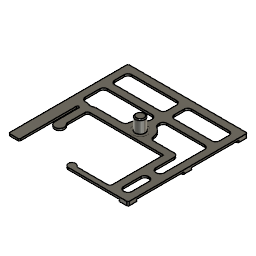
StentorCam Base (Autodesk Fusion 360 design; units mm, degrees)
Autodesk Fusion 360 part; units mm, degrees
note: some values were not read from the file. Set by a fixed rule: which sketch regions a step uses.
sketch "Sketch1" plane through (0, 0, 0) normal (0, 0, 1) x (1, 0, 0)
  line L0 (0, 0) -> (235, 0)
  line L1 (235, 0) -> (235, 235)
  line L2 (235, 235) -> (0, 235)
  line L3 (0, 235) -> (0, 0)
  line L4 (42.1, 114.8) -> (192.9, 114.8)
  line L5 (192.9, 114.8) -> (192.9, 10.2)
  line L6 (192.9, 10.2) -> (42.1, 10.2)
  line L7 (42.1, 10.2) -> (42.1, 114.8)
  line L8 (42.1, 114.8) -> (192.9, 10.2) construction
  line L9 (192.9, 114.8) -> (42.1, 10.2) construction
  circle A0 centre (125, 135) radius 10
  line L10 (125, 125) -> (117.5, 125) construction
  line L11 (117.5, 125) -> (117.5, 0) construction
  line L12 (-5, 240) -> (-5, -5)
  line L13 (-5, -5) -> (240, -5)
  line L14 (240, -5) -> (240, 240)
  line L15 (240, 240) -> (-5, 240)
  line L16 (117.5, 0) -> (117.5, -5) construction
  line L17 (110, -5) -> (125, -5)
  arc A1 (125, -5) -> (125, 0) centre (125, -2.5) ccw
  line L18 (125, 0) -> (110, 0)
  arc A2 (110, 0) -> (110, -5) centre (110, -2.5) ccw
  line L19 (110, -2.5) -> (125, -2.5) construction
  arc A3 (12.5, -5) -> (12.5, 0) centre (12.5, -2.5) ccw
  arc A4 (-2.5, 0) -> (-2.5, -5) centre (-2.5, -2.5) ccw
  arc A5 (237.5, -5) -> (237.5, 0) centre (237.5, -2.5) ccw
  arc A6 (222.5, 0) -> (222.5, -5) centre (222.5, -2.5) ccw
  line L20 (0, 117.5) -> (235, 117.5) construction
  circle A7 centre (125, 135) radius 15
  circle A8 centre (32.1, 62.5) radius 10
  line L21 (37.1, 62.5) -> (22.1, 62.5)
  line L22 (22.1, 62.5) -> (22.1, 114.8)
  line L23 (22.1, 114.8) -> (37.1, 114.8)
  line L24 (37.1, 114.8) -> (37.1, 62.5)
  line L25 (42.1, 114.8) -> (17.1, 114.8)
  line L26 (17.1, 114.8) -> (17.1, 10.2)
  line L27 (17.1, 10.2) -> (42.1, 10.2)
  line L28 (42.1, 10.2) -> (42.1, 114.8)
  circle A9 centre (117.5, 2.6) radius 7.6
  line L29 (117.5, -5) -> (17.1, -5)
  line L30 (17.1, -5) -> (17.1, 5.2)
  line L31 (17.1, 5.2) -> (117.5, 5.2)
  line L32 (117.5, 5.2) -> (117.5, -5)
  line L33 (192.9, 10.2) -> (17.1, 10.2)
  line L34 (17.1, 10.2) -> (17.1, 5.2)
  line L35 (17.1, 5.2) -> (192.9, 5.2)
  line L36 (192.9, 5.2) -> (192.9, 10.2)
  line L37 (192.9, 5.2) -> (192.9, -5)
  line L38 (17.1, 114.8) -> (-5, 114.8)
  arc A10 (235, -2.5) -> (240, -2.5) centre (237.5, -2.5) ccw
  arc A11 (240, 12.5) -> (235, 12.5) centre (237.5, 12.5) ccw
  arc A12 (235, 110) -> (240, 110) centre (237.5, 110) ccw
  arc A13 (240, 125) -> (235, 125) centre (237.5, 125) ccw
  arc A14 (235, 222.5) -> (240, 222.5) centre (237.5, 222.5) ccw
  arc A15 (240, 237.5) -> (235, 237.5) centre (237.5, 237.5) ccw
  arc A16 (237.5, 235) -> (237.5, 240) centre (237.5, 237.5) ccw
  arc A17 (222.5, 240) -> (222.5, 235) centre (222.5, 237.5) ccw
  arc A18 (125, 235) -> (125, 240) centre (125, 237.5) ccw
  arc A19 (110, 240) -> (110, 235) centre (110, 237.5) ccw
  arc A20 (12.5, 235) -> (12.5, 240) centre (12.5, 237.5) ccw
  arc A21 (-2.5, 240) -> (-2.5, 235) centre (-2.5, 237.5) ccw
  arc A22 (0, 237.5) -> (-5, 237.5) centre (-2.5, 237.5) ccw
  arc A23 (-5, 222.5) -> (0, 222.5) centre (-2.5, 222.5) ccw
  arc A24 (0, 125) -> (-5, 125) centre (-2.5, 125) ccw
  arc A25 (-5, 110) -> (0, 110) centre (-2.5, 110) ccw
  arc A26 (0, 12.5) -> (-5, 12.5) centre (-2.5, 12.5) ccw
  arc A27 (-5, -2.5) -> (0, -2.5) centre (-2.5, -2.5) ccw
  point P0 (125, 135)
  point P1 (117.5, 62.5)
  point P2 (117.5, -2.5)
  point P3 (117.5, 117.5)
  dimension "d1" = 235
  dimension "d2" = 235
  dimension "d3" = 125
  dimension "d4" = 135
  dimension "d6" = 104.6
  dimension "d7" = 150.8
  dimension "d8" = 20
  dimension "d9" = 5
  dimension "d10" = 15
  dimension "d13" = 112.5
  dimension "d14" = 0
  dimension "d22" = 30
  dimension "d36" = 20
  dimension "d37" = 5
  dimension "d39" = 15
  dimension "d41" = 5
  dimension "d43" = 360
  constraint horizontal L0
  constraint vertical L1
  constraint horizontal L2
  constraint vertical L3
  constraint coincident L0.start L3.end
  constraint horizontal L4
  constraint vertical L5
  constraint horizontal L6
  constraint vertical L7
  constraint midpoint L9 P1
  constraint coincident P0 A0.centre
  constraint coincident A0 L10.start
  constraint tangent A0 L10
  constraint midpoint L0 L11.end
  constraint perpendicular L0 L11
  constraint midpoint P1 L11
  constraint horizontal L10
  constraint midpoint L13 L16.end
  constraint tangent L17 A1
  constraint tangent A1 L18
  constraint parallel L17 L18
  constraint tangent L18 A2
  constraint tangent L17 A2
  constraint perpendicular L16 L19
  constraint midpoint L16 P2
  constraint midpoint L19 P2
  constraint coincident L0 A1.end
  constraint midpoint L3 L20.start
  constraint midpoint L1 L20.end
  constraint midpoint L20 P3
  constraint tangent L7 A8
  constraint horizontal L21
  constraint vertical L22
  constraint horizontal L23
  constraint vertical L24
  constraint tangent A8 L22
  constraint collinear L4 L23
  constraint horizontal L25
  constraint vertical L26
  constraint horizontal L27
  constraint vertical L28
  constraint coincident P1 L21
  constraint collinear L6 L27
  constraint coincident A8.centre L21
  constraint coincident L11 A9.centre
  constraint tangent L6 A9
  constraint tangent L13 A9
  constraint horizontal L29
  constraint vertical L30
  constraint horizontal L31
  constraint vertical L32
  constraint horizontal L33
  constraint vertical L34
  constraint horizontal L35
  constraint vertical L36
  constraint coincident L13 L37.end
  constraint perpendicular L13 L37
  constraint coincident L12 L38.end
  constraint perpendicular L12 L38
  measures "d1" distance of L0.start L0.end
  measures "d2" distance of L0.start L2.end
  measures "d3" distance of L3 P0
  measures "d4" distance of L0 P0
  measures "d6" distance of L4.start L6.end
  measures "d7" distance of L4.start L4.end
  measures "d8" diameter of A0
  measures "d10" distance of A2.centre A1.centre
  measures "d22" diameter of A7
  measures "d36" diameter of A8
  measures "d41" distance of L26.end L30.end
extrude "Extrude1" add sketch "Sketch1" along normal blind 4 contours L0 L3 L26 L30 L34 L38 | L0 L3 L12 L13 A3 A4 A26 A27 | L0 L13 A3 L30 | L3 L12 A25 A26 | L3 L12 L38 A25 | L3 L12 L38 A24 | L0 L1 L2 L3 L4 L5 L23 L25 L36 L37 L38 | L0 L18 A9 L31 L32 L35 | L0 L18 A9 L32 | A9 L31 L35 | L3 L12 A23 A24 | L0 L18 A9 L32 L35 | L0 L18 A9 L32 | L0 L13 L17 A1 L18 A9 | L2 L3 L12 L15 A20 A21 A22 A23 | A8 L22 L23 L24 L25 | L0 L18 A9 L35 L37 | L0 L13 A1 L37 | A8 L21 L24 | A8 L21 L24 | L0 L13 A6 L37 | L2 L15 A19 A20 | L12 L15 A21 A22 | L0 L1 L13 L14 A5 A6 A10 A11 | L2 L15 A18 A19 | L13 L14 A5 A10 | L2 L15 A17 A18 | L1 L2 L14 L15 A14 A15 A16 A17 | L1 L14 A11 A12 | L1 L14 A12 A13 | L1 L14 A13 A14 | L14 L15 A15 A16 | A7 makes body 1
extrude "Extrude4" add sketch "Sketch1" against normal blind 4 contours L3 L12 L38 A25 | L3 L12 L38 A24 | L2 L3 L12 L15 A20 A21 A22 A23 | L0 L1 L13 L14 A5 A6 A10 A11 | L2 L15 A18 A19 | L1 L2 L14 L15 A14 A15 A16 A17 | L1 L14 A12 A13 bodies 1
extrude "Extrude3" cut sketch "Sketch1" along normal blind 2.2 contours A7 bodies 1
ref_plane "WorkPlane1" through (117.5, 135, 2) normal (0, 1, 0) x (-1, 0, 0)
sketch "Sketch2" plane through (0, 135, 0) normal (0, 1, 0) x (1, 0, 0)
  line L0 (125, 0) -> (115, 0)
  line L1 (115, 0) -> (115, -30)
  line L2 (115, -30) -> (125, -30)
  line L3 (125, -30) -> (125, 0)
  line L4 (115, 0) -> (110, 0)
  line L5 (110, 0) -> (110, -2)
  line L6 (110, -2) -> (115, -2)
  line L7 (115, -2) -> (115, 0)
  point P0 (125, 0)
  dimension "d26" = 30
  dimension "d27" = 10
  dimension "d28" = 2
  dimension "d29" = 5
  constraint horizontal L0
  constraint vertical L1
  constraint horizontal L2
  constraint vertical L3
  constraint coincident P0 L0.start
  constraint horizontal L4
  constraint vertical L5
  constraint horizontal L6
  constraint vertical L7
  measures "d26" distance of P0 L2.end
  measures "d27" distance of L1.end L2.end
  measures "d28" distance of L4.end L5.end
  measures "d29" distance of L5.end L6.end
revolve "Revolve1" add sketch "Sketch2" angle 360 about axis through (125, 135, 30) along (0, 0, -1) separate body makes body 2 in component "Component"
fillet "Fillet3" radius 5 4 edges at (37.1, 114.8, 2) (192.9, 5.2, 2) (124.6414, 5.2, 2) (37.1, 71.1603, 2) on bodies 1
fillet "Fillet3" radius 2.5 2 edges at (17.1, 114.8, 2) (22.1, 114.8, 2) on bodies 1
fillet "Fillet4" radius 2.5 4 edges at (-5, 240, 2) (240, 240, 2) (240, -5, 2) (17.1, -5, 2) on bodies 1
move_face "OffsetFaces1" offset -0.2 2 faces at (134.9503, 134.0043, 2.8) (139.9255, 133.5065, 1.4667) on bodies 1
extrude "Extrude5" cut 1 faces at (138.4388, 133.7381, 2.2) along direction (0, 0, 1) blind 0.2 on bodies 1 bodies 1
chamfer "Chamfer1" distance 2 angle 45 1 edges at (115.6767, 138.6162, 30) on bodies 2 in component "Component"
sketch "Sketch3" plane through (0, 0, 4) normal (0, 0, 1) x (-1, 0, 0)
  arc A0 (-14.6, 5) -> (-17.1, 2.5) centre (-14.6, 2.5) ccw
  line L0 (-17.1, 2.5) -> (-17.1, -112.3)
  arc A1 (-22.1, -112.3) -> (-17.1, -112.3) centre (-19.6, -112.3) ccw
  line L1 (-22.1, -112.3) -> (-22.1, -62.5)
  arc A2 (-22.1, -62.5) -> (-38.7667, -69.9536) centre (-32.1, -62.5) ccw
  arc A3 (-37.1, -73.6803) -> (-38.7667, -69.9536) centre (-42.1, -73.6803) ccw
  line L2 (-37.1, -73.6803) -> (-37.1, -109.8)
  arc A4 (-42.1, -114.8) -> (-37.1, -109.8) centre (-42.1, -109.8) ccw
  line L3 (-42.1, -114.8) -> (-192.9, -114.8)
  line L4 (-192.9, -114.8) -> (-192.9, -10.2)
  arc A5 (-187.9, -5.2) -> (-192.9, -10.2) centre (-187.9, -10.2) ccw
  line L5 (-187.9, -5.2) -> (-127.5499, -5.2)
  arc A6 (-123.5618, -7.1841) -> (-127.5499, -5.2) centre (-127.5499, -10.2) ccw
  arc A7 (-123.5618, -7.1841) -> (-117.5, 5) centre (-117.5, -2.6) ccw
  line L6 (-117.5, 5) -> (-237.5, 5)
  arc A8 (-237.5, 5) -> (-240, 2.5) centre (-237.5, 2.5) ccw
  line L7 (-240, 2.5) -> (-240, -237.5)
  arc A9 (-240, -237.5) -> (-237.5, -240) centre (-237.5, -237.5) ccw
  line L8 (-237.5, -240) -> (2.5, -240)
  arc A10 (2.5, -240) -> (5, -237.5) centre (2.5, -237.5) ccw
  line L9 (5, -237.5) -> (5, 2.5)
  arc A11 (5, 2.5) -> (2.5, 5) centre (2.5, 2.5) ccw
  line L10 (2.5, 5) -> (-14.6, 5)
  circle A12 centre (-125, -135) radius 10.2
  line L11 (-225, -225) -> (-10, -225)
  line L12 (-10, -225) -> (-10, -126.9318)
  arc A13 (-30.4327, -126.0442) -> (-10, -126.9318) centre (-19.6, -112.3) ccw
  arc A14 (-42.1, -129.8) -> (-30.4327, -126.0442) centre (-42.1, -109.8) ccw
  line L13 (-42.1, -129.8) -> (-207.9, -129.8)
  line L14 (-207.9, -129.8) -> (-207.9, -10.2)
  arc A15 (-207.899, -10) -> (-207.9, -10.2) centre (-187.9, -10.2) ccw
  line L15 (-207.899, -10) -> (-225, -10)
  line L16 (-225, -10) -> (-225, -225)
  circle A16 centre (-125, -135) radius 25.2
  line L17 (-207.9, -76.2386) -> (-225, -76.2386)
  line L18 (-225, -76.2386) -> (-225, -61.2386)
  line L19 (-225, -61.2386) -> (-207.9, -61.2386)
  line L20 (-207.9, -61.2386) -> (-207.9, -76.2386)
  line L21 (-117.5, -225) -> (-132.5, -225)
  line L22 (-132.5, -225) -> (-132.5, -135)
  line L23 (-132.5, -135) -> (-117.5, -135)
  line L24 (-117.5, -135) -> (-117.5, -225)
  line L25 (-10, -189.8474) -> (-225, -189.8474)
  line L26 (-225, -189.8474) -> (-225, -174.8474)
  line L27 (-225, -174.8474) -> (-10, -174.8474)
  line L28 (-10, -174.8474) -> (-10, -189.8474)
  dimension "d57" = -15
  dimension "d58" = 15
  dimension "d59" = 15
  dimension "d60" = 15
  dimension "d61" = 15
  constraint horizontal L17
  constraint vertical L18
  constraint horizontal L19
  constraint vertical L20
  constraint coincident L16 L18.end
  constraint coincident L14 L17.start
  constraint horizontal L21
  constraint vertical L22
  constraint horizontal L23
  constraint vertical L24
  constraint coincident L11 L21.start
  constraint horizontal L25
  constraint vertical L26
  constraint horizontal L27
  constraint vertical L28
  constraint coincident L16 L26.end
  constraint coincident L12 L25.start
  constraint midpoint A12.centre L23
  measures "d59" distance of L25 L27
  measures "d60" distance of L22 L24
  measures "d61" distance of L17 L19
extrude "Extrude6" cut sketch "Sketch3" against normal blind 30 contours L12 A13 A14 L13 A16 L24 L27 | L13 L14 L16 A16 L17 L22 L27 | L14 A15 L15 L16 L19 | L11 L16 L22 L25 | L11 L12 L24 L25 bodies 1
fillet "Fillet5" radius 7.5 25 edges at (225, 225, 2) (225, 189.8474, 2) (132.5, 189.8474, 2) (132.5, 225, 2) (10, 225, 2) (117.5, 225, 2) (117.5, 189.8474, 2) (10, 189.8474, 2) (100.3423, 129.8, 2) (117.5, 159.0581, 2) (117.5, 174.8474, 2) (10, 174.8474, 2) (10, 126.9318, 2) (149.6577, 129.8, 2) (132.5, 159.0581, 2) (132.5, 174.8474, 2) (225, 174.8474, 2) (225, 76.2386, 2) (207.9, 76.2386, 2) (225, 61.2386, 2) (207.9, 61.2386, 2) (225, 10, 2) (207.899, 10, 2) (30.4327, 126.0442, 2) (207.9, 129.8, 2) on bodies 1
component "Component" placed x (1, 0, 0) y (0, 1, 0) z (0, 0, 1) at (0, 0, 0)
equation "d6 = 105.6 mm - 1 mm"
equation "d7 = 151.8 mm - 1 mm"
